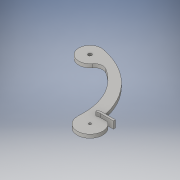
# Autodesk Inventor part: Part2
Saved by Autodesk Inventor 2016 (Build 200138000, 138)
## iProperties
Created: 2016-01-12
Part Number: Part2
Material: Generic
Document SubType Name: Modeling
Designer: cemer
Density: 1 g/cm^3
Appearance: Default
Author: cemer
Autodesk Inventor part; units mm, degrees
ref_plane "YZ Plane" through (0, 0, 0) normal (1, 0, 0) x (0, 1, 0)
ref_plane "XZ Plane" through (0, 0, 0) normal (0, 1, 0) x (-1, 0, 0)
ref_plane "XY Plane" through (0, 0, 0) normal (0, 0, 1) x (1, 0, 0)
sketch "Sketch1" plane through (0, 0, 0) normal (0, 1, 0) x (-1, 0, 0)
  circle A0 centre (0, 0) radius 11.43
  circle A1 centre (0, 0) radius 9.525
  dimension "d0" = 22.86
  dimension "d1" = 19.05
  constraints: 2 centre point, 2 coincident
  measures "d0" diameter of A0
  measures "d1" diameter of A1
extrude "Extrusion1" add sketch "Sketch1" along normal blind 6.35
sketch "Sketch2" plane through (0, 6.35, 0) normal (0, 1, 0) x (1, 0, 0)
  circle A0 centre (0, 0) radius 11.43
  constraints: 1 centre point, 1 coincident
extrude "Extrusion2" add sketch "Sketch2" along normal blind 3.175
sketch "Sketch3" plane through (0, 9.525, 0) normal (0, 1, 0) x (1, 0, 0)
  circle A0 centre (0, 0) radius 1.1
  dimension "d6" = 2.2
  constraints: 1 centre point, 1 coincident
  measures "d6" diameter of A0
extrude "Extrusion3" cut sketch "Sketch3" against normal blind 7.9375
sketch "Sketch6" plane through (0, 0, 0) normal (0, -1, 0) x (1, 0, 0)
  line L0 (-16.0948, 0) -> (0, 0)
  line L1 (0, 0) -> (0, -15.3841)
  line L2 (0, -15.3841) -> (-16.0948, -15.3841)
  line L3 (-16.0948, -15.3841) -> (-16.0948, 0)
  line L4 (-16.0948, 14.6504) -> (12.3807, 14.6504)
  line L5 (12.3807, 14.6504) -> (12.3807, -15.3841)
  line L6 (12.3807, -15.3841) -> (-16.0948, -15.3841)
  line L7 (-16.0948, -15.3841) -> (-16.0948, 14.6504)
  constraints: 16 end point, 4 parallel, 2 horizontal, 2 perpendicular
extrude "Extrusion6" cut sketch "Sketch6" against normal blind 6.35 contours L7 L4 L5 L6 L1 L0
sketch "Sketch7" plane through (0, 0, -9.525) normal (1, 0, 0) x (0, 0, -1)
  line L0 (1.905, 6.35) -> (-20.955, 6.35) projected
  line L1 (1.905, 6.35) -> (0, 6.35)
  line L2 (0, 6.35) -> (0, 0)
  line L3 (0, 0) -> (1.905, 0)
  line L4 (1.905, 0) -> (1.905, 6.35)
  point P0 (-9.525, 0)
  point P1 (-9.525, 6.35)
  constraints: 8 end point, 2 parallel, 1 horizontal, 1 perpendicular
extrude "Extrusion7" add sketch "Sketch7" along normal blind 11.43
sketch "Sketch8" plane through (0, 0, 0) normal (0, -1, 0) x (1, 0, 0)
  line L0 (0, 0) -> (-10.5625, -10.5625)
  line L1 (0, 0) -> (14.9376, 0) construction
  line L2 (-10.5625, -10.5625) -> (-17.6997, 3.3244)
  line L3 (-17.6997, 3.3244) -> (0, 0)
  dimension "d18" = 135
  constraints: 8 end point, 1 equal length, 1 horizontal
  measures "d18" angle of L0 L1
extrude "Extrusion8" cut sketch "Sketch8" against normal blind 6.35
sketch "Sketch9" plane through (0, 0, 0) normal (0, -1, 0) x (1, 0, 0)
  line L0 (0, 0) -> (-6.0166, -14.5254)
  line L1 (0, 0) -> (15.7222, 0) construction
  line L2 (-6.0166, -14.5254) -> (-13.1372, -7.2627)
  line L3 (-13.1372, -7.2627) -> (0, 0)
  dimension "d21" = 112.5
  constraints: 8 end point, 1 equal length, 1 horizontal
  measures "d21" angle of L0 L1
extrude "Extrusion9" cut sketch "Sketch9" against normal blind 6.35
sketch "Sketch13" plane through (0, 9.525, 0) normal (0, 1, 0) x (1, 0, 0)
  line L0 (0, 0) -> (-53.8815, 53.8815)
  line L1 (0, 0) -> (76.2, 0) construction
  circle A0 centre (-53.8815, 53.8815) radius 10.16
  arc A1 (6.3182, 9.525) -> (0, 11.43) centre (0, 0) ccw projected
  line L2 (0, 11.43) -> (0, 53.8815)
  line L3 (0, 53.8815) -> (-50.1886, 63.3466)
  arc A2 (-4.3741, 10.5599) -> (6.3182, 9.525) centre (0, 0) ccw projected
  line L4 (-11.43, 0) -> (-11.43, 42.4515)
  line L5 (-11.43, 42.4515) -> (-43.7215, 53.8815)
  circle A3 centre (-53.8815, 53.8815) radius 1.65
  circle A4 centre (0, 0) radius 1.1 projected
  circle A5 centre (0, 0) radius 1.65
  dimension "d44" = 76.2
  dimension "d45" = 135
  dimension "d46" = 20.32
  dimension "d47" = 100.68
  dimension "d48" = 3.3
  dimension "d49" = 3.3
  constraints: 12 end point, 3 centre point, 3 coincident, 3 point on circle, 2 vertical, 1 equal length, 1 horizontal, 1 tangent
  measures "d44" distance of L0.start L0.end
  measures "d45" angle of L1 L0
  measures "d46" diameter of A0
  measures "d47" angle of L3 L2
  measures "d48" diameter of A3
  measures "d49" diameter of A5
extrude "Extrusion13" add sketch "Sketch13" against normal blind 3.175 contours A2 L4 L0 | L0 L4 L5 A0 L3 L2 A1 A2 | A0
fillet "Fillet3" radius 50.8 1 edges at (-11.43, 7.9375, -42.4515)
fillet "Fillet4" radius 7.62 1 edges at (-43.7215, 7.9375, -53.8815)
fillet "Fillet5" radius 63.5 1 edges at (0, 7.9375, -53.8815)
mirror "Mirror1" about plane through (0, 6.35, -11.43) normal (0, 1, 0) of "Extrusion1", "Extrusion7"
sketch "Sketch14" plane through (0, 12.7, -11.43) normal (0, 1, 0) x (1, 0, 0)
  line L0 (0, -11.43) -> (-4.3741, -0.8701)
  line L1 (-4.3741, -0.8701) -> (-16.9777, -0.8701)
  line L2 (-16.9777, -0.8701) -> (-16.9777, -27.9599)
  line L3 (-16.9777, -27.9599) -> (23.6628, -27.9599)
  line L4 (0, -1.905) -> (11.43, -1.905) projected
  line L5 (23.6628, -27.9599) -> (11.43, -1.905)
  line L6 (11.43, -1.905) -> (0, -1.905)
  line L7 (0, -1.905) -> (0, -11.43)
  constraints: 14 end point, 3 perpendicular, 1 collinear, 1 horizontal
extrude "Extrusion14" cut sketch "Sketch14" against normal blind 3.175
sketch "Sketch15" plane through (0, 6.35, 0) normal (0, -1, 0) x (1, 0, 0)
  line L0 (-24.6585, 25.4032) -> (37.4015, 25.4032)
  line L1 (37.4015, 25.4032) -> (37.4015, -39.3047)
  line L2 (37.4015, -39.3047) -> (-24.6585, -39.3047)
  line L3 (-24.6585, -39.3047) -> (-24.6585, 25.4032)
  point P0 (0, 0)
  constraints: 8 end point, 2 parallel, 1 horizontal, 1 perpendicular
extrude "Extrusion15" cut sketch "Sketch15" along normal blind 26.9875
body "Solid1"
